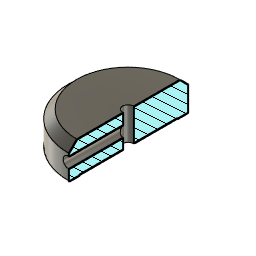
BearingPadRound (Autodesk Fusion 360 design; units mm, degrees)
Autodesk Fusion 360 part; units mm, degrees
sketch "Sketch1" plane through (0, 0, 0) normal (0, 0, 1) x (1, 0, 0)
  circle A0 centre (0, 0) radius 11
  dimension "d1" = 22
  constraint coincident A0.centre origin
  measures "d1" diameter of A0
extrude "Extrude1" add sketch "Sketch1" along normal blind 6
chamfer "Chamfer1" distance 1.5 angle 45 1 edges at (-10.2556, -3.9778, 6)
fillet "Fillet1" radius 0.1 1 edges at (-10.2556, -3.9778, 0)
sketch "Sketch2" plane through (0, 0, 0) normal (0, 0, -1) x (1, 0, 0)
  circle A0 centre (0, 0) radius 10.9
  circle A1 centre (0, 0) radius 1
  dimension "d7" = 2
  constraint concentric A0 A1
  measures "d7" diameter of A1
extrude "Extrude2" cut sketch "Sketch2" against normal blind 10 contours A1
sketch "Sketch3" plane through (0, 0, 0) normal (0, 1, 0) x (1, 0, 0)
  circle A0 centre (0, -3) radius 1
  dimension "d10" = 2
  dimension "d11" = 3
  measures "d10" diameter of A0
  measures "d11" distance of origin A0.centre
extrude "Extrude3" cut sketch "Sketch3" against normal blind 19
sketch "Sketch4" plane through (0, 0, 0) normal (0, 0, -1) x (1, 0, 0)
  circle A0 centre (0, 0) radius 1
  circle A1 centre (0, 0) radius 10.9
  circle A2 centre (0, 0) radius 9
  dimension "d14" = 18
  constraint coincident A0.centre A1.centre
  measures "d14" diameter of A2
extrude "Extrude4" cut sketch "Sketch4" against normal blind 0.1 thin wall 0.1 centred open curves A2
sketch "Sketch5" plane through (0, 0, 0) normal (0, 0, -1) x (1, 0, 0)
  circle A0 centre (0, 0) radius 8.95
  circle A1 centre (0, 0) radius 1
  line L0 (-9, 0) -> (9, 0)
  constraint horizontal L0
extrude "Extrude5" cut sketch "Sketch5" against normal blind 0.1 thin wall 0.1 centred open curves L0
pattern_circular "C-Pattern1" count 2 over 90 about axis through (0, 0, 1.75) along (0, 0, 1) of "Extrude5"
